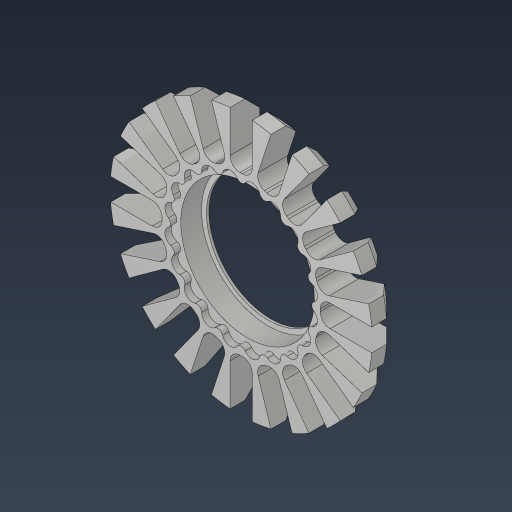
# Autodesk Inventor part: Raddeckel Getriebe
Saved by Autodesk Inventor 2023.1 (Build 271208000, 208)
## iProperties
Part Number: Raddeckel Getriebe
Material: Aluminium 6061
Document SubType Name: Modeling
Designer: rYan
Mass: 12.1113 g
Surface Area: 49.3887 cm^2
Volume: 4.48568 cm^3
Density: 2.7 g/cm^3
Appearance: Aluminium - flach
Author: rYan
Autodesk Inventor part; units mm, degrees
ref_plane "YZ Plane" through (0, 0, 0) normal (1, 0, 0) x (0, 1, 0)
ref_plane "XZ Plane" through (0, 0, 0) normal (0, 1, 0) x (-1, 0, 0)
sketch "Skizze1" plane through (0, 0, 0) normal (0, 0, 1) x (1, 0, 0)
  line L0 (0, 0) -> (0, 4)
  line L1 (26.5, 6) -> (26.5, 0)
  line L2 (26.5, 0) -> (15.6, 0)
  line L3 (13.515, 1.3) -> (13.515, 5.5)
  line L4 (13.515, 1.3) -> (15.6, 1.3)
  line L5 (15.6, 1.3) -> (15.6, 0)
  line L6 (13.515, 5.5) -> (12.515, 5.5)
  line L7 (12.515, 5.5) -> (12.515, 6)
  line L8 (12.515, 6) -> (26.5, 6)
  dimension "d1" = 27.03
  dimension "d2" = 53
  dimension "d4" = 6
  dimension "d25" = 31.2
  dimension "d52" = 1
  dimension "d53" = 0.5
  dimension "d54" = 4.2
  constraints: 18 end point, 6 perpendicular, 1 horizontal, 1 point on line, 1 vertical
  measures "d1" diameter of L3 L0
  measures "d2" diameter of L1 L0
  measures "d4" distance of L1.start L1.end
  measures "d25" diameter of L5 L0
  measures "d52" distance between parallel lines of L7 L3
  measures "d53" distance of L6.end L7.end
  measures "d54" distance of L3.start L3.end
revolve "Umdrehung1" add sketch "Skizze1" angle 360 about axis through (0, 0, 0) along (0, 1, 0)
ref_plane "Arbeitsebene1" through (0, 6, 0) normal (0, 1, 0) x (1, 0, 0)
chamfer "Fase2" distance 3 angle 45 1 edges at (-26.5, 6, 0)
sketch "Skizze2" plane through (0, 0, 0) normal (0, 1, 0) x (-1, 0, 0)
  circle A0 centre (0, 0) radius 16 construction
  circle A1 centre (0, 0) radius 26.5 projected
  line L0 (0, 0) -> (0, 26.5) construction
  line L1 (2.25, 26.5) -> (-2.25, 26.5)
  line L2 (-2.25, 26.5) -> (-2.25, 18)
  line L3 (-0.25, 16) -> (0.25, 16)
  line L4 (2.25, 18) -> (2.25, 26.5)
  arc A2 (0.25, 16) -> (2.25, 18) centre (0.25, 18) ccw
  arc A3 (-2.25, 18) -> (-0.25, 16) centre (-0.25, 18) ccw
  point P0 (-2.25, 16)
  point P1 (2.25, 16)
  dimension "d6" = 32
  dimension "d7" = 4.5
  dimension "d8" = 2
  constraints: 10 end point, 5 tangent, 4 point on circle, 4 point on line, 3 centre point, 2 parallel, 1 coincident, 1 equal radius, 1 horizontal, 1 midpoint, 1 perpendicular, 1 vertical, 1 vertical alignment, 2 other
  measures "d6" diameter of A0
  measures "d7" distance of point (-2.25, 16) point (2.25, 16)
  measures "d8" radius of A2
extrude "Extrusion1" cut sketch "Skizze2" along normal through all contours L4 A2 L3 A3 L2 A1 | A1 L1 L4 | L2 L1 A1 picked at (0, 20.833333)
pattern_circular "Runde Anordnung1" count 20 over 360 about axis through (0, -10, 0) along (0, 1, 0) of "Extrusion1"
sketch "Skizze9" plane through (0, 0, 0) normal (0, 1, 0) x (-1, 0, 0)
  circle A0 centre (0, 0) radius 15.6
  circle A1 centre (0, 0) radius 14.3 construction
  line L0 (0, 0) -> (2.440378, -15.407938) construction
  line L1 (0, -21.887738) -> (0, 21.847956) construction
  arc A2 (-2.440378, -15.407938) -> (-0.816651, -14.722868) centre (-2.179345, -13.759845) ccw
  arc A3 (0.816651, -14.722868) -> (-0.816651, -14.722868) centre (0, -15.3) ccw
  arc A4 (0.816651, -14.722868) -> (2.440378, -15.407938) centre (2.179345, -13.759845) ccw
  dimension "d55" = 31.2
  dimension "d57" = 9
  dimension "d58" = 1
  dimension "d59" = 1.66864
  dimension "d65" = 15.3
  constraints: 8 point on circle, 5 tangent, 4 centre point, 2 end point, 1 coincident, 1 other
  measures "d55" diameter of A0
  measures "d57" angle of L0 L1
  measures "d58" radius of A3
  measures "d59" radius of A4
  measures "d65" distance of point (0, 0) A3.centre
extrude "Extrusion5" add sketch "Skizze9" along normal up to surface (1.3 mm away) contours A2 A3 A4 A0 picked at (0, -15.152414)
pattern_circular "Runde Anordnung2" count 20 over 360 about axis through (0, -10, 0) along (0, 1, 0) of "Extrusion5"
